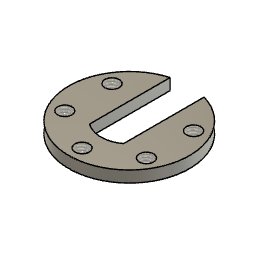
cryo clamp upper v8 (Autodesk Fusion 360 design; units mm, degrees)
Autodesk Fusion 360 part; units mm, degrees
note: some values were not read from the file. Set by a fixed rule: which sketch regions a step uses; the direction of a hole.
sketch "Sketch1" plane through (0, 0, 0) normal (0, 1, 0) x (1, 0, 0)
  circle A0 centre (0, 0) radius 16
  circle A1 centre (0, 0) radius 7.5
  line L0 (-4.5, 15.3542) -> (-4.5, -6)
  line L1 (4.5, -6) -> (4.5, 15.3542)
  circle A2 centre (0, 0) radius 12.5 construction
  point P0 (0, -12.5)
  dimension "d1" = 32
  dimension "d2" = 15
  dimension "d3" = 9
  dimension "d4" = 25
  constraint coincident A0.centre A1.centre
  constraint coincident A0 L0.start
  constraint coincident A1 L0.end
  constraint vertical L0
  constraint coincident A1 L1.start
  constraint coincident A0 L1.end
  constraint parallel L0 L1
  constraint horizontal L0.end L1.start
  constraint concentric A1 A2
  constraint coincident A2 P0
  constraint vertical A0.centre P0
  measures "d1" diameter of A0
  measures "d2" diameter of A1
  measures "d3" distance of L0 L1
  measures "d4" diameter of A2
extrude "Extrude1" add sketch "Sketch1" along normal blind 3 contours A0 A1 L0 L1 | A1 L1 | A1 L0 picked at (10.3483, -8.0939) makes body 1
hole "Hole1" at (0, 0, 12.5) direction (0, 1, 0) diameter 3.783 end through all bodies 1
thread "Thread2" "ISO Metric profile 4.5 M4.5x0.75 6H" thread offset 0 thread depth 10
pattern_circular "C-Pattern1" count 6 over 360 about axis through (0, 1.75, 0) along (0, 1, 0) of "Hole1"
extrude "Extrude2" add sketch "Sketch1" along normal blind 3 separate body makes body 2
hole "Hole2" at (0, 0, 12.5) direction (0, 1, 0) diameter 4.5 depth 3 tip angle 118 bodies 2
pattern_circular "C-Pattern2" count 6 over 360 about axis through (0, 1.75, 0) along (0, 1, 0) of "Hole2"
hole "Hole3" at (0, 0, 0) direction (0, 1, 0) diameter 2 end through all bodies 2
copy_body "Body->Comp1" bodies 1 removing the originals makes body 3 in component "LC"
copy_body "Body->Comp2" bodies 2 removing the originals makes body 4 in component "UC"
sketch "Sketch2" plane through (0, 3, 0) normal (0, 1, 0) x (-1, 0, 0)
  circle A0 centre (0, 0) radius 1
  circle A1 centre (10.8253, 6.25) radius 2.25
  circle A2 centre (10.8253, -6.25) radius 2.25
  circle A3 centre (0, -12.5) radius 2.25
  circle A4 centre (-10.8253, -6.25) radius 2.25
  circle A5 centre (-10.8253, 6.25) radius 2.25
  circle A6 centre (0, 12.5) radius 2.25
  circle A7 centre (0, 0) radius 16
sketch "Sketch3" plane through (0, 3, 0) normal (0, 1, 0) x (-1, 0, 0)
  circle A0 centre (10.8253, 6.25) radius 1.8916
  circle A1 centre (10.8253, -6.25) radius 1.8916
  circle A2 centre (-10.8253, -6.25) radius 1.8915
  circle A3 centre (-10.8253, 6.25) radius 1.8915
  circle A4 centre (0, 12.5) radius 1.8916
  arc A5 (4.5, -15.3542) -> (-4.5, -15.3542) centre (0, 0) ccw
  line L0 (-4.5, -15.3542) -> (-4.5, 6)
  arc A6 (4.5, 6) -> (-4.5, 6) centre (0, 0) ccw
  line L1 (4.5, 6) -> (4.5, -15.3542)
component "LC" placed x (1, 0, 0) y (0, 1, 0) z (0, 0, 1) at (0, 0, 0)
component "UC" placed x (1, 0, 0) y (0, 1, 0) z (0, 0, 1) at (0, 0, 0)
named bodies: "LC", "UC"
